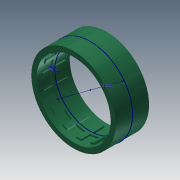
# Autodesk Inventor part: Tire
Saved by Autodesk Inventor 2015 (Build 190159000, 159)
## iProperties
Created: 2016-11-10
Part Number: Tire
Material: ABS Plastic
Document SubType Name: Modeling
Designer: Aniket Pant
Density: 1.06 g/cm^3
Appearance: Smooth - Dark Sea Green
Author: Aniket Pant
Autodesk Inventor part; units mm, degrees
ref_plane "YZ Plane" through (0, 0, 0) normal (1, 0, 0) x (0, 1, 0)
ref_plane "XZ Plane" through (0, 0, 0) normal (0, 1, 0) x (-1, 0, 0)
sketch "Sketch2" plane through (0, 0, 0) normal (0, 0, 1) x (1, 0, 0)
  circle A0 centre (0, 0) radius 20.955
  circle A1 centre (0, 0) radius 18.415
  circle A2 centre (0, 0) radius 17.653
  dimension "d4" = 41.91
  dimension "d5" = 2.54
  dimension "d6" = 0.762
  constraints: 3 centre point, 1 coincident
  measures "d4" diameter of A0
  measures "d5" radial gap between concentric circles of A0 A1
  measures "d6" radial gap between concentric circles of A1 A2
extrude "Extrusion2" add sketch "Sketch2" along normal mid plane 16.51 contours A0
ref_plane "Work Plane1" through (0, 0, 0) normal (0, 0, 1) x (1, 0, 0)
sketch "Sketch4" plane through (0, 0, 0) normal (0, 0, 1) x (1, 0, 0)
  line L0 (0, 0) -> (0, 18.3729) construction
  circle A0 centre (0, 0) radius 18.415 projected
  circle A1 centre (0, 0) radius 17.653 projected
  line L1 (1.2314, 17.61) -> (1.2846, 18.3701)
  circle A2 centre (0, 0) radius 18.415 projected
  line L2 (-1.2314, 17.61) -> (-1.2846, 18.3701)
  dimension "d11" = 4
  dimension "d12" = 4
  constraints: 6 end point, 6 point on circle, 1 vertical
  measures "d11" angle of L0 L2
  measures "d12" angle of L0 L1
extrude "Extrusion3" add sketch "Sketch4" along normal mid plane 11.43 contours L1 A1 L2 A0 picked at (-0.1369, 18.1561)
pattern_circular "Circular Pattern1" count 16 over 360 about axis through (0, 0, 0) along (0, 0, 1) of "Extrusion3"
extrude "Extrusion4" add sketch "Sketch2" along normal blind 1.27 contours A1
body "Solid2"
